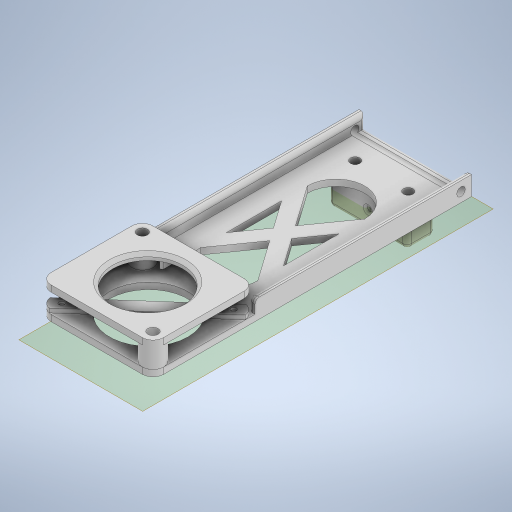
# Autodesk Inventor part: CableSupport-Knomi
Saved by Autodesk Inventor 2023 (Build 270158000, 158)
## iProperties
Created: 2024-03-22
Part Number: CableSupport-Knomi
Material: Generic
Document SubType Name: Modeling
Designer: incep
Density: 1 g/cm^3
Appearance: Default
Author: incep
## iProperties of the stored document CableSupport-Knomi_3DPrint.ipt
Created: 2024-03-22
Part Number: CableSupport-Knomi_3DPrint
Material: Generic
Document SubType Name: Modeling
Designer: incep
Density: 1 g/cm^3
Appearance: Default
Author: incep
Autodesk Inventor part; units mm, degrees
ref_plane "YZ Plane" through (0, 0, 0) normal (1, 0, 0) x (0, 1, 0)
ref_plane "XZ Plane" through (0, 0, 0) normal (0, 1, 0) x (-1, 0, 0)
sketch "Sketch1" plane through (0, 0, 0) normal (0, 1, 0) x (-1, 0, 0)
  line L0 (21.5, -19) -> (-21.5, -19) construction
  line L1 (-21.5, -19) -> (-21.5, 19) construction
  line L2 (-21.5, 19) -> (21.5, 19) construction
  line L3 (21.5, 19) -> (21.5, -19) construction
  circle A0 centre (21.5, -19) radius 2.4
  circle A1 centre (-21.5, 19) radius 2.4
  line L4 (26.5, -126) -> (-26.5, -126)
  line L5 (-26.5, -126) -> (-26.5, 24)
  line L6 (-26.5, 24) -> (26.5, 24)
  line L7 (26.5, 24) -> (26.5, -126)
  point P0 (0, 0)
  point P1 (0, -19)
  point P2 (-21.5, 0)
  point P3 (0, 19)
  point P4 (0, 24)
  dimension "d0" = 43
  dimension "d1" = 38
  dimension "d2" = 4.8
  dimension "d3" = 5
  dimension "d4" = 5
  dimension "d5" = 150
  constraints: 16 end point, 4 midpoint, 4 parallel, 2 centre point, 2 coincident, 2 horizontal, 2 perpendicular, 2 vertical alignment, 1 equal radius, 1 horizontal alignment
  measures "d0" distance of L0.start L0.end
  measures "d1" distance of L0.end L1.end
  measures "d2" diameter of A0
  measures "d3" distance between parallel lines of L5 L1
  measures "d4" distance between parallel lines of L6 L2
  measures "d5" distance of L4.end L5.end
extrude "Extrusion1" add sketch "Sketch1" along normal blind 3
sketch "Sketch2" plane through (0, 3, 0) normal (0, 1, 0) x (1, 0, 0)
  line L0 (-26.5, -24) -> (26.5, -24) projected
  line L1 (26.5, -24) -> (26.5, 126) projected
  line L2 (26.5, 126) -> (-26.5, 126) projected
  line L3 (-26.5, 126) -> (-26.5, -24) projected
  circle A0 centre (21.5, -19) radius 2.4 projected
  circle A1 centre (-21.5, 19) radius 2.4 projected
  line L4 (23.5, 123) -> (23.5, -21)
  line L5 (23.5, -21) -> (-23.5, -21)
  line L6 (-23.5, -21) -> (-23.5, 123)
  line L7 (-23.5, 123) -> (23.5, 123)
  line L8 (-23.5, 123) -> (-23.5, 126)
  line L9 (23.5, 123) -> (23.5, 126)
  line L10 (-23.5, 24) -> (-26.5, 24)
  line L11 (23.5, 24) -> (26.5, 24)
  point P0 (0, 0)
  point P1 (-25, 24)
  dimension "d8" = 3
  dimension "d9" = 5
  constraints: 16 end point, 8 point on line, 3 perpendicular, 1 midpoint, 3 other
  measures "d8" distance between parallel lines of L1 L4
  measures "d9" vertical distance of point (-25, 24) A1.centre
extrude "Extrusion2" add sketch "Sketch2" along normal blind 6 contours L3 L2 L8 L6 L10 | L11 L4 L9 L2 L1
sketch "Sketch3" plane through (-26.5, 0, -126) normal (-1, 0, 0) x (0, 0, 1)
  circle A0 centre (5, 4.5) radius 2
  line L0 (0, 0) -> (0, 9) projected
  point P0 (126, 0)
  point P1 (0, 4.5)
  dimension "d12" = 4
  dimension "d13" = 5
  constraints: 1 centre point, 1 horizontal alignment, 1 midpoint
  measures "d12" diameter of A0
  measures "d13" distance from line of L0 A0.centre
extrude "Extrusion3" cut sketch "Sketch3" against normal up to surface (53 mm away)
fillet "Fillet1" radius 2 5 edges at (0, 3, -126) (23.5, 6, -126) (-23.5, 6, -126) (-23.5, 9, -75) (23.5, 9, -75)
fillet "Fillet2" radius 2 6 edges at (-24.0858, 8.4142, -24) (-23.5, 5, -24) (-26, 9, -24) (26, 9, -24) (23.5, 5, -24) (24.0858, 8.4142, -24)
fillet "Fillet3" radius 5 2 edges at (-26.5, 1.5, 24) (26.5, 1.5, 24)
sketch "Sketch4" plane through (0, 0, 0) normal (0, -1, 0) x (1, 0, 0)
  circle A0 centre (1.4992, 1.0001) radius 18.4992 projected
  point P0 (0, 0)
extrude "Extrusion4" cut sketch "Sketch4" against normal up to surface (3 mm away)
sketch "Sketch5" plane through (0, 3, 0) normal (0, 1, 0) x (1, 0, 0)
  line L0 (-1, 24) -> (1, 24)
  line L1 (1, 24) -> (1, -24)
  line L2 (1, -24) -> (-1, -24)
  line L3 (-1, -24) -> (-1, 24)
  line L4 (-21.5, -24) -> (21.5, -24) projected
  point P0 (0, 0)
  point P1 (0, 24)
  point P2 (1, 0)
  dimension "d21" = 2
  constraints: 8 end point, 2 midpoint, 2 parallel, 1 collinear, 1 horizontal, 1 horizontal alignment, 1 perpendicular, 1 vertical alignment
  measures "d21" distance of L0.start L0.end
extrude "Extrusion5" [suppressed]
sketch "Sketch6" plane through (0, 3, 0) normal (0, 1, 0) x (1, 0, 0)
  circle A0 centre (1.4992, -1.0001) radius 18.4992 projected
  circle A1 centre (-21.5, 19) radius 2.4 projected
  circle A2 centre (21.5, -19) radius 2.4 projected
  arc A3 (21.5, -24) -> (26.5, -19) centre (21.5, -19) ccw projected
  line L0 (26.5, -19) -> (26.5, 24) projected
  line L1 (26.5, 24) -> (25.5, 24) projected
  arc A4 (23.5, 26) -> (25.5, 24) centre (25.5, 26) ccw projected
  line L2 (23.5, 26) -> (23.5, 119.6771) projected
  line L3 (23.5, 119.6771) -> (-23.5, 119.6771) projected
  line L4 (-23.5, 119.6771) -> (-23.5, 26) projected
  arc A5 (-25.5, 24) -> (-23.5, 26) centre (-25.5, 26) ccw projected
  line L5 (-25.5, 24) -> (-26.5, 24) projected
  line L6 (-26.5, 24) -> (-26.5, -19) projected
  arc A6 (-26.5, -19) -> (-21.5, -24) centre (-21.5, -19) ccw projected
  line L7 (-21.5, -24) -> (21.5, -24) projected
  circle A7 centre (-21.5, 19) radius 5
  circle A8 centre (21.5, -19) radius 2.4 projected
  circle A9 centre (21.5, -19) radius 5
  point P0 (0, 0)
  dimension "d25" = 10
  constraints: 2 centre point, 2 coincident, 1 equal radius
  measures "d25" diameter of A7
extrude "Extrusion7" add sketch "Sketch6" along normal blind 9 separate body contours A9 A3 | A7
sketch "Sketch7" plane through (-21.5, 12, -19) normal (0, 1, 0) x (1, 0, 0)
  circle A0 centre (0, 0) radius 5 projected
  circle A1 centre (0, 0) radius 2.4 projected
  circle A2 centre (43, -38) radius 5 projected
  circle A3 centre (43, -38) radius 2.4 projected
  line L0 (0, 0) -> (43, -38) construction
  circle A4 centre (22.9992, -20.0001) radius 18.4992 projected
  circle A5 centre (0, 0) radius 2.4 projected
  circle A6 centre (43, -38) radius 2.4 projected
  arc A7 (43, -43) -> (48, -38) centre (43, -38) ccw projected
  line L1 (48, -38) -> (48, 5) projected
  line L2 (48, 5) -> (47, 5) projected
  arc A8 (45, 7) -> (47, 5) centre (47, 7) ccw projected
  line L3 (45, 7) -> (45, 100.6771) projected
  line L4 (45, 100.6771) -> (-2, 100.6771) projected
  line L5 (-2, 100.6771) -> (-2, 7) projected
  arc A9 (-4, 5) -> (-2, 7) centre (-4, 7) ccw projected
  line L6 (-4, 5) -> (-5, 5) projected
  line L7 (-5, 5) -> (-5, -38) projected
  arc A10 (-5, -38) -> (0, -43) centre (0, -38) ccw projected
  line L8 (0, -43) -> (43, -43) projected
  line L9 (48, 5) -> (-5, 5)
  circle A11 centre (21.5, -19) radius 16.5
  point P0 (0, 5)
  point P1 (-5, 0)
  point P2 (48, -38)
  dimension "d30" = 33
  constraints: 4 end point, 1 centre point, 1 coincident, 1 collinear
  measures "d30" diameter of A11
extrude "Extrusion8" add sketch "Sketch7" along normal blind 3 contours A0 | A0 L9 L2 L1 A2 L8 A10 L7 | A2 | A4 bodies 2
chamfer "Chamfer1" distance 1.5 angle 45 1 edges at (-16.5, 15, 0)
fillet "Fillet4" radius 5 1 edges at (26.5, 13.5, -24)
ref_plane "Work Plane1" through (-21.5, 5, -19) normal (0, -1, 0) x (1, 0, 0)
sketch "Sketch8" plane through (-21.5, 5, -19) normal (0, -1, 0) x (1, 0, 0)
  arc A0 (43, -5) -> (48, 0) centre (43, 0) ccw projected
  line L0 (48, 38) -> (48, 0) projected
  arc A1 (43, 43) -> (48, 38) centre (43, 38) ccw projected
  line L1 (0, 43) -> (43, 43) projected
  arc A2 (0, 43) -> (-5, 38) centre (0, 38) ccw projected
  line L2 (-5, 0) -> (-5, 38) projected
  arc A3 (0, -5) -> (-5, 0) centre (0, 0) ccw projected
  line L3 (43, -5) -> (0, -5) projected
  circle A4 centre (21.5, 19) radius 16.5 projected
  circle A5 centre (43, 0) radius 1.25
  circle A6 centre (0, 38) radius 1.25
  line L4 (51.0219, -11.0927) -> (54.9951, -6.5968)
  line L5 (54.9951, -6.5968) -> (-9.0126, 49.9682)
  line L6 (-9.0126, 49.9682) -> (-12.9858, 45.4723)
  line L7 (-12.9858, 45.4723) -> (51.0219, -11.0927)
  line L8 (43, 0) -> (0, 38) construction
  point P0 (-10.9992, 47.7203)
  point P1 (-4.9839, 38.4008)
  point P2 (44.0107, -4.8968)
  point P3 (47.9839, -0.4008)
  point P4 (-1.0107, 42.8968)
  dimension "d38" = 2.5
  dimension "d39" = 6
  constraints: 10 end point, 3 parallel, 2 centre point, 2 coincident, 1 equal radius, 1 midpoint, 1 perpendicular, 1 point on line
  measures "d38" diameter of A5
  measures "d39" distance between parallel lines of L5 L7
extrude "Extrusion9" add sketch "Sketch8" along normal blind 2 separate body contours L7 A4 L5 A0 | L7 A4 L5 | L7 A2 L5 A4
sketch "Sketch9" plane through (-21.5, 3, -19) normal (0, -1, 0) x (1, 0, 0)
  circle A0 centre (0, 38) radius 1.25 projected
  circle A1 centre (43, 0) radius 1.25 projected
  circle A2 centre (0, 38) radius 1.25 projected
  circle A3 centre (0, 38) radius 2.25
  circle A4 centre (43, 0) radius 2.25
  point P0 (21.5, 19)
  dimension "d42" = 4.5
  constraints: 2 centre point, 2 coincident, 1 equal radius
  measures "d42" diameter of A3
extrude "Extrusion10" cut sketch "Sketch9" against normal blind 1 contours A0 | A1 | A3 | A4 bodies 3
sketch "Sketch10" plane through (-21.5, 12, -19) normal (0, -1, 0) x (1, 0, 0)
  circle A0 centre (0, 38) radius 1.25 projected
  circle A1 centre (43, 0) radius 1.25 projected
  circle A2 centre (0, 38) radius 1.75
  circle A3 centre (43, 0) radius 1.75
  point P0 (21.5, 19)
  dimension "d45" = 3.5
  constraints: 2 centre point, 2 coincident, 1 equal radius
  measures "d45" diameter of A2
extrude "Extrusion11" cut sketch "Sketch10" against normal blind 2.5 contours A0 | A1 | A2 | A3 bodies 2
sketch "Sketch11" plane through (-21.5, 12, -19) normal (0, -1, 0) x (1, 0, 0)
  circle A0 centre (21.5, 19) radius 16.5 projected
  circle A1 centre (21.5, 19) radius 18.16
  circle A2 centre (21.5, 19) radius 19.16
  line L0 (12.09, 16.687) -> (30.91, 16.687)
  line L1 (30.91, 16.687) -> (30.91, -3.36)
  line L2 (30.91, -3.36) -> (12.09, -3.36)
  line L3 (12.09, -3.36) -> (12.09, 16.687)
  line L4 (7.107, 37.16) -> (35.6246, 37.16) construction
  line L5 (31.91, -4.36) -> (31.91, 17.687)
  line L6 (31.91, 17.687) -> (11.09, 17.687)
  line L7 (11.09, 17.687) -> (11.09, -4.36)
  line L8 (11.09, -4.36) -> (31.91, -4.36)
  point P0 (21.5, 16.687)
  point P1 (11.09, 2.9147)
  point P2 (11.09, 4.1199)
  point P3 (31.91, 4.1199)
  point P4 (31.91, 2.9147)
  point P5 (30.91, 3.4682)
  point P6 (30.91, 2.31)
  point P7 (12.09, 2.31)
  point P8 (12.09, 3.4682)
  dimension "d48" = 36.32
  dimension "d49" = 1
  dimension "d50" = 18.82
  dimension "d51" = 40.52
  dimension "d52" = 1
  constraints: 18 end point, 4 parallel, 2 centre point, 2 horizontal, 2 perpendicular, 1 coincident, 1 midpoint, 1 tangent, 1 vertical alignment, 3 other
  measures "d48" diameter of A1
  measures "d49" radial gap between concentric circles of A1 A2
  measures "d50" distance of L0.start L0.end
  measures "d51" distance between parallel lines of L2 L4
  measures "d52" distance between parallel lines of L1 L5
extrude "Extrusion12" add sketch "Sketch11" along normal blind 1 contours L7 A2 L5 A1 | A1 L3 A2 L7 | L5 A2 L1 A1 bodies 2
extrude "Extrusion13" add sketch "Sketch11" along normal blind 5 contours A2 L3 L2 L1 L5 L8 L7 bodies 2
sketch "Sketch13" plane through (0, 0, 0) normal (0, -1, 0) x (1, 0, 0)
  line L0 (12.5, -110.1771) -> (-12.5, -110.1771) construction
  line L1 (18.5, -116.6771) -> (-18.5, -116.6771)
  line L2 (-18.5, -116.6771) -> (-18.5, -103.6771)
  line L3 (-18.5, -103.6771) -> (18.5, -103.6771)
  line L4 (18.5, -103.6771) -> (18.5, -116.6771)
  line L5 (26.5, -126) -> (-26.5, -126) construction
  line L6 (-23.5, -119.6771) -> (-23.5, -122.3229) construction
  line L7 (23.5, -119.6771) -> (-23.5, -119.6771) construction
  line L8 (23.5, -122.3229) -> (23.5, -119.6771) construction
  line L9 (-23.5, -122.3229) -> (23.5, -122.3229) construction
  line L10 (26.5, -119) -> (26.5, -123) construction
  line L11 (-26.5, -123) -> (-26.5, -119) construction
  circle A0 centre (12.5, -110.1771) radius 2.8
  circle A1 centre (-12.5, -110.1771) radius 2.8
  circle A2 centre (12.5, -110.1771) radius 2.25
  circle A3 centre (-12.5, -110.1771) radius 2.25
  point P0 (0, 0)
  point P1 (0, -110.1771)
  point P2 (-18.5, -110.1771)
  point P3 (0, -116.6771)
  point P4 (18.5, -110.1771)
  dimension "d58" = 25
  dimension "d59" = 13
  dimension "d61" = 3
  dimension "d62" = 5.6
  dimension "d63" = 5.6
  dimension "d64" = 6
  dimension "d65" = 4.5
  dimension "d66" = 4.5
  constraints: 10 end point, 4 centre point, 4 coincident, 4 midpoint, 2 horizontal, 2 parallel, 2 vertical alignment, 1 horizontal alignment, 1 perpendicular
  measures "d58" distance of L0.start L0.end
  measures "d59" distance between parallel lines of L3 L1
  measures "d61" distance between parallel lines of L7 L1
  measures "d62" diameter of A0
  measures "d63" diameter of A1
  measures "d64" distance of point (18.5, -110.177) L0.start
  measures "d65" diameter of A2
  measures "d66" diameter of A3
extrude "Extrusion14" cut sketch "Sketch13" against normal up to surface (3 mm away) contours A2 | A3 bodies 1
extrude "Extrusion15" add sketch "Sketch13" along normal blind 15 separate body contours L1 L2 L3 L4
ref_plane "Work Plane2" through (0, -7.5, 0) normal (0, -1, 0) x (1, 0, 0)
sketch "Sketch14" plane through (0, -7.5, 0) normal (0, -1, 0) x (1, 0, 0)
  line L0 (18.5, -103.6771) -> (-18.5, -103.6771) projected
  line L1 (-18.5, -103.6771) -> (-18.5, -116.6771) projected
  line L2 (-18.5, -116.6771) -> (18.5, -116.6771) projected
  line L3 (18.5, -116.6771) -> (18.5, -103.6771) projected
  circle A0 centre (-12.5, -110.1771) radius 2.8 projected
  circle A1 centre (12.5, -110.1771) radius 2.8 projected
  line L4 (2.25, -116.6771) -> (-2.25, -116.6771)
  line L5 (-2.25, -116.6771) -> (-2.25, -103.6771)
  line L6 (-2.25, -103.6771) -> (2.25, -103.6771)
  line L7 (2.25, -103.6771) -> (2.25, -116.6771) construction
  line L8 (3.25, -116.6771) -> (-3.25, -116.6771)
  line L9 (-3.25, -116.6771) -> (-3.25, -114.1771)
  line L10 (-3.25, -114.1771) -> (3.25, -114.1771) construction
  line L11 (3.25, -114.1771) -> (3.25, -116.6771)
  line L12 (4, -114.1771) -> (-4, -114.1771) construction
  line L13 (-4, -114.1771) -> (-4, -108.1771)
  line L14 (-4, -108.1771) -> (4, -108.1771) construction
  line L15 (4, -108.1771) -> (4, -114.1771)
  line L16 (3.25, -114.1771) -> (4, -112.4771)
  line L17 (2.25, -103.6771) -> (1.2, -103.6771)
  line L18 (1.2, -103.6771) -> (1.2, -105.6771)
  line L19 (1.2, -105.6771) -> (2.25, -105.6771)
  line L20 (2.25, -105.6771) -> (2.25, -103.6771)
  line L21 (0, -116.6771) -> (0, -103.6771)
  line L22 (2.25, -108.1771) -> (2.25, -105.6771)
  line L23 (4, -108.1771) -> (2.25, -108.1771)
  point P0 (0, 0)
  point P1 (0, -114.1771)
  dimension "d71" = 4.5
  dimension "d72" = 6.5
  dimension "d73" = 2.5
  dimension "d74" = 6
  dimension "d75" = 8
  dimension "d76" = 1.7
  dimension "d77" = 1.2
  dimension "d78" = 2
  constraints: 40 end point, 8 parallel, 7 midpoint, 4 horizontal, 4 perpendicular, 3 point on line, 2 collinear, 1 vertical
  measures "d71" distance between parallel lines of L5 L7
  measures "d72" distance of L8.start L8.end
  measures "d73" distance of L8.end L9.end
  measures "d74" distance of L12.end L13.end
  measures "d75" distance of L12.start L12.end
  measures "d76" distance from line of L16.end L12
  measures "d77" distance of L17.end L21.end
  measures "d78" distance of L17.end L18.end
revolve "Revolution1" cut sketch "Sketch14" angle 360 about axis through (0, -7.5, -116.6771) along (0, 0, 1) bodies 4 contours L18 L19 L22 L23 L15 L16 L11 L2 L21 L0
chamfer "Chamfer2" distance 1 angle 45 1 edges at (-3.25, -7.5, -116.6771)
fillet "Fillet5" radius 1 1 edges at (-1.2, -7.5, -103.6771)
fillet "Fillet6" radius 2 8 edges at (18.5, -7.5, -103.6771) (18.5, -15, -110.1771) (18.5, -7.5, -116.6771) (0, -15, -116.6771) (0, -15, -103.6771) (-18.5, -15, -110.1771) (-18.5, -7.5, -103.6771) (-18.5, -7.5, -116.6771)
sketch "Sketch15" plane through (0, 3, 0) normal (0, 1, 0) x (1, 0, 0)
  line L0 (0, 88.6771) -> (0, 38.36) construction
  line L1 (-13.5, 88.6771) -> (-13.5, 38.36)
  line L2 (13.5, 38.36) -> (13.5, 88.6771)
  arc A0 (13.5, 88.6771) -> (-13.5, 88.6771) centre (0, 88.6771) ccw
  arc A1 (-13.5, 38.36) -> (13.5, 38.36) centre (0, 38.36) ccw
  line L3 (16.5, 103.6771) -> (-16.5, 103.6771) projected
  line L4 (-10.41, 23.36) -> (10.41, 23.36) projected
  line L5 (-23.5, 26) -> (-23.5, 124) projected
  line L6 (-13.5, 76.5512) -> (13.5, 38.36)
  line L7 (-13.5, 88.6771) -> (13.5, 50.4859)
  line L8 (13.5, 88.6771) -> (-13.5, 50.4859)
  line L9 (-13.5, 38.36) -> (13.5, 76.5512)
  point P0 (0, 0)
  point P1 (0, 63.5186)
  point P2 (0, 57.4556)
  point P3 (4.2863, 63.5186)
  point P4 (-4.2863, 63.5186)
  point P5 (0, 69.5815)
  dimension "d85" = 15
  dimension "d86" = 15
  dimension "d87" = 10
  dimension "d88" = 7
  dimension "d89" = 7
  dimension "d90" = 13.5
  constraints: 16 end point, 4 point on circle, 4 point on line, 4 tangent, 3 parallel, 2 centre point, 1 midpoint, 1 vertical
  measures "d85" distance from line of L0.start L3
  measures "d86" distance from line of L4 L0.end
  measures "d87" distance between parallel lines of L5 L1
  measures "d88" distance between parallel lines of L7 L6
  measures "d89" distance between parallel lines of L9 L8
  measures "d90" radius of A0
extrude "Extrusion16" cut sketch "Sketch15" against normal up to surface (3 mm away) contours A0 L8 L7 | L6 L8 L1 | L2 L7 L9 | L9 L6 A1 bodies 1
body "Solid1"
body "Solid2"
body "Solid3"
body "Solid4"
body "Solid5"
